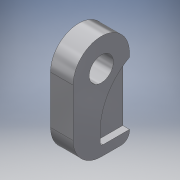
# Autodesk Inventor part: Soporte-Disipador
Saved by Autodesk Inventor 2018.3 (Build 223284000, 284)
## iProperties
Created: 2021-05-06
Part Number: Soporte-Disipador
Material: Genérico
Document SubType Name: Modeling
Designer: laguerre
Density: 8.47 g/cm^3
Appearance: Suave - Blanco
Author: laguerre
Autodesk Inventor part; units mm, degrees
ref_plane "YZ Plane" through (0, 0, 0) normal (1, 0, 0) x (0, 1, 0)
ref_plane "XZ Plane" through (0, 0, 0) normal (0, 1, 0) x (-1, 0, 0)
ref_plane "XY Plane" through (0, 0, 0) normal (0, 0, 1) x (1, 0, 0)
sketch "Boceto39" plane through (0, 0, 0) normal (0, 0, 1) x (1, 0, 0)
  circle A0 centre (0, 0) radius 2.15
  line L0 (-5, 5) -> (0, 5)
  line L1 (5, 0) -> (5, -13.5)
  line L2 (5, -13.5) -> (-5, -13.5)
  line L3 (-5, -13.5) -> (-5, 5)
  arc A1 (5, 0) -> (0, 5) centre (0, 0) ccw
  dimension "d373" = 4.3
  dimension "d374" = 5
  dimension "d375" = 10
  dimension "d376" = 18.5
  constraints: 8 end point, 2 centre point, 2 coincident, 2 parallel, 2 point on circle, 2 tangent, 1 horizontal, 1 perpendicular
  measures "d373" diameter of A0
  measures "d374" radius of A1
  measures "d375" distance between parallel lines of L1 L3
  measures "d376" distance between parallel lines of L0 L2
extrude "Extrusión13" add sketch "Boceto39" along normal blind 4
sketch "Boceto40" plane through (-5, -13.5, 0) normal (-1, 0, 0) x (0, 0, 1)
  line L0 (0, 0) -> (0, 18.5) construction
  line L1 (0, 0) -> (4, 0) construction
  line L2 (4, 18.5) -> (4, 0) construction
  line L3 (0, 18.5) -> (4, 18.5) construction
  line L4 (0, 4) -> (1.2, 4)
  line L5 (1.2, 4) -> (1.2, 1.7)
  line L6 (1.2, 1.7) -> (0, 1.7)
  line L7 (0, 1.7) -> (0, 4)
  line L8 (4, 18.5) -> (4, 0) projected
  line L9 (4, 4) -> (2.8, 4)
  line L10 (2.8, 4) -> (2.8, 1.7)
  line L11 (2.8, 1.7) -> (4, 1.7)
  line L12 (4, 1.7) -> (4, 4)
  point P0 (0, 13.5)
  dimension "d379" = 1.7
  dimension "d380" = 2.3
  dimension "d381" = 1.2
  constraints: 16 end point, 4 parallel, 4 point on line, 2 horizontal, 2 perpendicular, 1 collinear
  measures "d379" distance between parallel lines of L6 L1
  measures "d380" distance of L4.end L5.end
  measures "d381" distance of L5.end L6.end
extrude "Extrusión14" cut sketch "Boceto40" against normal blind 5.2
sketch "Boceto41" plane through (0, 0, 0) normal (0, 0, -1) x (-1, 0, 0)
  line L0 (-0.2, -11.8) -> (-0.2, -9.5) construction
  line L1 (5, -9.5) -> (5, 5) construction
  arc A0 (5, -0.7273) -> (-0.2, -9.5) centre (9.8, -9.5) ccw
  line L2 (5, 5) -> (5, -9.5) construction
  line L3 (-0.2, -9.5) -> (5, -9.5)
  line L4 (5, -9.5) -> (5, -0.7273)
  point P0 (0, 0)
  dimension "d384" = 10
  constraints: 4 end point, 3 point on circle, 2 point on line, 1 centre point, 1 horizontal, 1 tangent
  measures "d384" radius of A0
extrude "Extrusión15" cut sketch "Boceto41" against normal up to surface (1.2 mm away)
sketch "Boceto42" plane through (0, 0, 4) normal (0, 0, 1) x (1, 0, 0)
  line L0 (-5, -9.5) -> (0.2, -9.5) projected
  line L1 (0.2, -9.5) -> (0.2, -11.8) construction
  line L2 (0.2, -11.8) -> (-5, -11.8) construction
  line L3 (-5, -11.8) -> (-5, -13.5) construction
  line L4 (-5, -13.5) -> (5, -13.5) construction
  line L5 (5, -13.5) -> (5, 0) construction
  arc A0 (5, 0) -> (0, 5) centre (0, 0) ccw construction
  line L6 (0, 5) -> (-5, 5) construction
  line L7 (-5, 5) -> (-5, -9.5) construction
  circle A1 centre (0, 0) radius 2.15 construction
  line L8 (-5, -0.7273) -> (-5, -11.8) construction
  arc A2 (0.2, -9.5) -> (-5, -0.7273) centre (-9.8, -9.5) ccw projected
  line L9 (0.2, -9.5) -> (0.2, -11.8) construction
  line L10 (-5, -11.8) -> (0.2, -11.8) construction
  line L11 (-5, -11.8) -> (-5, -9.5) projected
  line L12 (-5, -9.5) -> (-5, -0.7273)
  line L13 (-5, -9.5) -> (0.2, -9.5) projected
  line L14 (-5, -9.5) -> (0.2, -9.5)
  line L15 (0.2, -9.5) -> (0.2, -11.8) projected
  line L16 (-5, -0.7273) -> (-5, -11.8) projected
  arc A3 (0.2, -9.5) -> (-5, -0.7273) centre (-9.8, -9.5) ccw
  constraints: 4 end point, 2 point on circle, 1 centre point, 1 collinear, 1 concentric, 1 horizontal
extrude "Extrusión16" cut sketch "Boceto42" against normal up to surface (1.2 mm away)
fillet "Empalme44" radius 5 1 edges at (-5, 5, 2)
fillet "Empalme45" radius 5 1 edges at (5, -13.5, 2)
fillet "Empalme46" radius 1.5 1 edges at (-5, -13.5, 2)
fillet "Empalme46" radius 0.5 2 edges at (0.2, -11.8, 0.6) (0.2, -11.8, 3.4)
